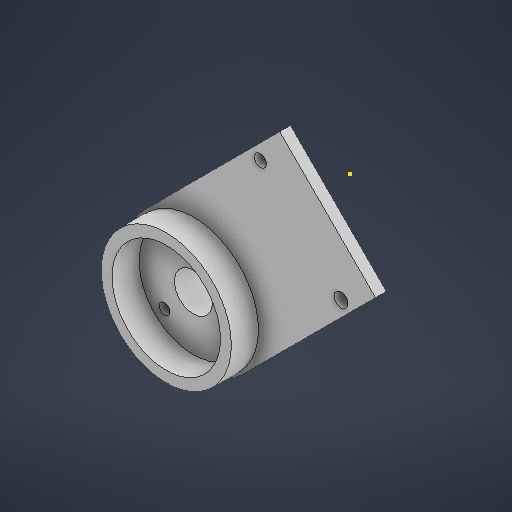
# Autodesk Inventor part: motorbracket
Saved by Autodesk Inventor 2027 (Build 310192000, 192)
## iProperties
Created: 2026-06-29
Part Number: motorbracket
Material: Generic
Document SubType Name: Modeling
Designer: uchiha
Density: 1 g/cm^3
Appearance: Default
Author: uchiha
Autodesk Inventor part; units mm, degrees
ref_plane "YZ Plane" through (0, 0, 0) normal (1, 0, 0) x (0, 1, 0)
ref_plane "XZ Plane" through (0, 0, 0) normal (0, 1, 0) x (-1, 0, 0)
ref_plane "XY Plane" through (0, 0, 0) normal (0, 0, 1) x (1, 0, 0)
sketch "Sketch1" plane through (0, 0, 0) normal (0, 0, 1) x (1, 0, 0)
  circle A0 centre (-26.8226, -31.265) radius 3.5
  arc A1 (-35.6614, -22.4261) -> (-17.9837, -40.1038) centre (-26.8226, -31.265) ccw
  circle A2 centre (38.1774, 33.735) radius 1.5
  circle A3 centre (-14.4482, -4.0414) radius 1
  circle A4 centre (0.401, -18.8906) radius 1
  line L0 (-14.4482, -4.0414) -> (0.401, -18.8906)
  line L1 (-17.9837, -40.1038) -> (-35.6614, -22.4261)
  line L2 (-35.6614, -22.4261) -> (-10.9127, 2.3226)
  line L3 (-35.6614, -22.4261) -> (-10.9127, 2.3226)
  line L4 (-10.9127, 2.3226) -> (6.765, -15.3551)
  line L5 (6.765, -15.3551) -> (-17.9837, -40.1038)
  circle A5 centre (-14.4482, -4.0414) radius 1.127
  circle A6 centre (0.401, -18.8906) radius 1.2923
  circle A7 centre (0.401, -18.8906) radius 1.0598
  line L6 (-26.8226, -31.265) -> (-2.0738, -6.5162)
  line L7 (37.1168, 32.6744) -> (38.1774, 33.735)
  point P0 (0, 0)
  point P1 (38.1774, -31.265)
  dimension "d0" = 35
  constraints: 16 end point, 7 centre point, 3 perpendicular, 2 midpoint, 2 point on circle, 1 coincident, 1 tangent, 3 other
  measures "d0" distance of L2.end L1.end
extrude "Extrusion1" add sketch "Sketch1" along normal blind 2 contours A0 L6 L4 L5 L1 | A0 L1 L2 L4 L6 | L1 A1 A0
sketch "Sketch2" plane through (0, 0, 2) normal (0, 0, 1) x (1, 0, 0)
  circle A0 centre (-26.8226, -31.265) radius 3.5 projected
  circle A1 centre (-26.8226, -31.265) radius 10
  circle A2 centre (-26.8226, -31.265) radius 12
  point P0 (0, 0)
  dimension "d3" = 20
  dimension "d4" = 2
  constraints: 2 centre point
  measures "d3" diameter of A1
  measures "d4" radial gap between concentric circles of A1 A2
extrude "Extrusion2" add sketch "Sketch2" along normal blind 5 contours A2
sketch "Sketch3" plane through (0, 0, 0) normal (0, 0, -1) x (-1, 0, 0)
  line L0 (-6.765, -15.3551) -> (10.9127, 2.3226) projected
  line L1 (2.0738, -6.5162) -> (35.766, -40.2084)
  circle A0 centre (26.8226, -31.265) radius 3.5 projected
  arc A1 (17.9837, -40.1038) -> (35.6614, -22.4261) centre (26.8226, -31.265) ccw projected
  line L2 (26.8226, -31.265) -> (17.9837, -40.1038)
  circle A2 centre (32.1259, -36.5683) radius 1
  circle A3 centre (28.7637, -24.0205) radius 1
  circle A4 centre (19.5781, -33.2061) radius 1
  point P0 (0, 0)
  dimension "d7" = 2
  dimension "d8" = 15
  dimension "d11" = 360
  constraints: 4 end point, 3 centre point, 1 midpoint, 1 perpendicular, 1 point on line, 7 other
  measures "d7" diameter of A2
  measures "d8" diameter of A2.centre L2
extrude "Extrusion3" cut sketch "Sketch3" against normal blind 5 contours A2 L1 | L1 A2 | A3 | A4
sketch "Sketch4" plane through (0, 0, 0) normal (0, 0, -1) x (-1, 0, 0)
  circle A0 centre (32.1259, -36.5683) radius 1 projected
  circle A1 centre (19.5781, -33.2061) radius 1 projected
  circle A2 centre (28.7637, -24.0205) radius 1 projected
  line L0 (17.9837, -40.1038) -> (-6.765, -15.3551) projected
  arc A3 (17.9837, -40.1038) -> (35.6614, -22.4261) centre (26.8226, -31.265) ccw projected
  line L1 (10.9127, 2.3226) -> (35.6614, -22.4261) projected
  line L2 (-6.765, -15.3551) -> (10.9127, 2.3226) projected
  circle A4 centre (14.4482, -4.0414) radius 1.127 projected
  circle A5 centre (-0.401, -18.8906) radius 1.2923 projected
  circle A6 centre (26.8226, -31.265) radius 3.5 projected
  circle A7 centre (26.8226, -31.265) radius 4.5
  point P0 (0, 0)
  dimension "d15" = 1
  constraints: 1 centre point
  measures "d15" radial gap between concentric circles of A6 A7
extrude "Extrusion4" add sketch "Sketch4" along normal blind 5 contours A7
sketch "Sketch5" plane through (0, 0, 0) normal (1, 0, 0) x (0, 1, 0)
  point P0 (0, 0)
sketch "Sketch6" plane through (0, 0, 0) normal (0, 0, -1) x (-1, 0, 0)
  point P0 (0, 0)
body "Solid1"
